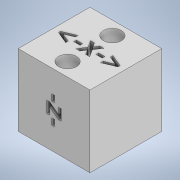
# Autodesk Inventor part: squareCalibrationBlock-1in
Saved by Autodesk Inventor 2021 (Build 250183000, 183)
## iProperties
Created: 2020-06-02
Part Number: squareCalibrationBlock-1in
Material: Generic
Document SubType Name: Modeling
Designer: robst
Density: 1 g/cm^3
Appearance: Default
Author: robst
Autodesk Inventor part; units mm, degrees
ref_plane "YZ Plane" through (0, 0, 0) normal (1, 0, 0) x (0, 1, 0)
ref_plane "XZ Plane" through (0, 0, 0) normal (0, 1, 0) x (-1, 0, 0)
ref_plane "XY Plane" through (0, 0, 0) normal (0, 0, 1) x (1, 0, 0)
sketch "Sketch1" plane through (0, 0, 0) normal (0, 1, 0) x (-1, 0, 0)
  line L0 (12.7, 12.7) -> (-12.7, 12.7)
  line L1 (-12.7, 12.7) -> (-12.7, -12.7)
  line L2 (-12.7, -12.7) -> (12.7, -12.7)
  line L3 (12.7, -12.7) -> (12.7, 12.7)
  line L4 (12.7, 12.7) -> (-12.7, -12.7) construction
  line L5 (-12.7, 12.7) -> (12.7, -12.7) construction
  point P0 (0, 0)
  dimension "d0" = 25.4
  dimension "d1" = 25.4
  constraints: 12 end point, 2 midpoint, 2 parallel, 1 horizontal, 1 perpendicular
  measures "d0" distance of L0.start L0.end
  measures "d1" distance of L1.end L0.end
extrude "Extrusion1" add sketch "Sketch1" along normal blind 25.4
sketch "Sketch2" plane through (0, 25.4, 0) normal (0, 1, 0) x (1, 0, 0)
  line L0 (-12.7, 12.7) -> (-12.7, -12.7) construction
  line L1 (-12.7, 0) -> (12.7, 0) construction
  line L2 (12.7, -12.7) -> (12.7, 12.7) construction
  line L3 (-6.1256, -2.4906) -> (-10.5058, -0.671)
  line L4 (-10.5058, -0.671) -> (-10.5058, 0.0782)
  line L5 (-10.5058, 0.0782) -> (-6.1256, 1.8978)
  line L6 (-6.1256, 1.8978) -> (-6.1256, 0.9551)
  line L7 (-6.1256, 0.9551) -> (-9.1885, -0.3005)
  line L8 (-9.1885, -0.3005) -> (-6.1256, -1.5479)
  line L9 (-6.1256, -1.5479) -> (-6.1256, -2.4906)
  line L10 (-2.7705, -0.7698) -> (-5.0306, -0.7698)
  line L11 (-5.0306, -0.7698) -> (-5.0306, 0.177)
  line L12 (-5.0306, 0.177) -> (-2.7705, 0.177)
  line L13 (-2.7705, 0.177) -> (-2.7705, -0.7698)
  line L14 (2.433, -2.54) -> (0.9592, -2.54)
  line L15 (0.9592, -2.54) -> (-0.0206, -0.9221)
  line L16 (-0.0206, -0.9221) -> (-1.0209, -2.54)
  line L17 (-1.0209, -2.54) -> (-2.433, -2.54)
  line L18 (-2.433, -2.54) -> (-0.7822, 0.0165)
  line L19 (-0.7822, 0.0165) -> (-2.3671, 2.54)
  line L20 (-2.3671, 2.54) -> (-0.8933, 2.54)
  line L21 (-0.8933, 2.54) -> (0.0247, 1.0045)
  line L22 (0.0247, 1.0045) -> (0.9674, 2.54)
  line L23 (0.9674, 2.54) -> (2.3794, 2.54)
  line L24 (2.3794, 2.54) -> (0.7863, 0.07)
  line L25 (0.7863, 0.07) -> (2.433, -2.54)
  line L26 (5.1088, -0.7698) -> (2.8488, -0.7698)
  line L27 (2.8488, -0.7698) -> (2.8488, 0.177)
  line L28 (2.8488, 0.177) -> (5.1088, 0.177)
  line L29 (5.1088, 0.177) -> (5.1088, -0.7698)
  line L30 (10.5881, -0.671) -> (6.208, -2.4906)
  line L31 (6.208, -2.4906) -> (6.208, -1.5479)
  line L32 (6.208, -1.5479) -> (9.2667, -0.2964)
  line L33 (9.2667, -0.2964) -> (6.208, 0.9551)
  line L34 (6.208, 0.9551) -> (6.208, 1.8978)
  line L35 (6.208, 1.8978) -> (10.5881, 0.0782)
  line L36 (10.5881, 0.0782) -> (10.5881, -0.671)
  point P0 (0, 0)
  constraints: 2 end point, 2 midpoint, 1 horizontal
extrude "Extrusion2" cut sketch "Sketch2" against normal blind 5.08
sketch "Sketch3" plane through (-12.7, 0, 12.7) normal (0, 0, 1) x (1, 0, 0)
  line L0 (12.6794, 25.4) -> (11.6791, 25.4) construction
  line L1 (12.7, 0) -> (12.6794, 25.4) construction
  line L2 (11.9178, 15.2517) -> (11.916, 17.5118)
  line L3 (11.916, 17.5118) -> (12.8628, 17.5126)
  line L4 (12.8628, 17.5126) -> (12.8647, 15.2525)
  line L5 (12.8647, 15.2525) -> (11.9178, 15.2517)
  line L6 (10.1514, 10.6602) -> (10.1481, 14.6863)
  line L7 (10.1481, 14.6863) -> (11.0991, 14.6871)
  line L8 (11.0991, 14.6871) -> (14.2626, 12.3472)
  line L9 (14.2626, 12.3472) -> (14.2608, 14.5661)
  line L10 (14.2608, 14.5661) -> (15.2282, 14.5669)
  line L11 (15.2282, 14.5669) -> (15.2312, 10.8001)
  line L12 (15.2312, 10.8001) -> (14.2638, 10.7994)
  line L13 (14.2638, 10.7994) -> (11.1168, 13.131)
  line L14 (11.1168, 13.131) -> (11.1188, 10.661)
  line L15 (11.1188, 10.661) -> (10.1514, 10.6602)
  line L16 (11.9238, 7.8911) -> (11.922, 10.1511)
  line L17 (11.922, 10.1511) -> (12.8688, 10.1519)
  line L18 (12.8688, 10.1519) -> (12.8706, 7.8918)
  line L19 (12.8706, 7.8918) -> (11.9238, 7.8911)
  constraints: 2 end point, 1 other
extrude "Extrusion3" cut sketch "Sketch3" against normal blind 5.08
sketch "Sketch11" plane through (0, 25.4, 0) normal (0, 1, 0) x (1, 0, 0)
  circle A0 centre (0, 7.9375) radius 3.175
  circle A1 centre (0, -7.9375) radius 3.175
  line L0 (12.7, 12.7) -> (-12.7, 12.7) projected
  line L1 (-12.7, -12.7) -> (12.7, -12.7) projected
  point P0 (0, 0)
  dimension "d81" = 6.35
  dimension "d82" = 4.7625
  dimension "d83" = 4.7625
  constraints: 2 centre point, 1 equal radius
  measures "d81" diameter of A0
  measures "d82" distance from line of A0.centre L0
  measures "d83" distance from line of A1.centre L1
extrude "Extrusion4" cut sketch "Sketch11" against normal blind 25.4
equation "\"d46\" = 0.125 * Sketch7_Pitch"
equation "\"Sketch7_Pitch\" = 1.27"
equation "\"d48\" = 60deg"
equation "\"d67\" = 0.125 * Sketch9_Pitch"
equation "\"Sketch9_Pitch\" = 1.27"
equation "\"d69\" = 60deg"
equation "\"d99\" = 0.125 * Sketch12_Pitch"
equation "\"Sketch12_Pitch\" = 1.27"
equation "\"d101\" = 60deg"
equation "\"d120\" = 0.125 * Sketch14_Pitch"
equation "\"Sketch14_Pitch\" = 1.27"
equation "\"d122\" = 60deg"
equation "\"d143\" = 55deg"
equation "\"Sketch16_Pitch\" = 1.27"
equation "\"d161\" = 55deg"
equation "\"Sketch18_Pitch\" = 1.27"
body "Solid1"
